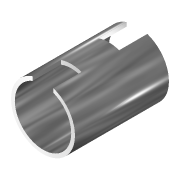
# Autodesk Inventor part: Pernament magnet
Saved by Autodesk Inventor 2020.3 (Build 243373010, 373A)
## iProperties
Created: 2021-04-26
Part Number: Pernament magnet
Material: Stainless Steel AISI 304
Document SubType Name: Modeling
Designer: marti
Density: 8 g/cm^3
Appearance: Chrome - Satin
Author: marti
Autodesk Inventor part; units mm, degrees
ref_plane "YZ Plane" through (0, 0, 0) normal (1, 0, 0) x (0, 1, 0)
ref_plane "XZ Plane" through (0, 0, 0) normal (0, 1, 0) x (-1, 0, 0)
ref_plane "XY Plane" through (0, 0, 0) normal (0, 0, 1) x (1, 0, 0)
sketch "Sketch1" plane through (0, 0, 0) normal (0, 0, 1) x (1, 0, 0)
  circle A0 centre (0, 0) radius 7.5
  circle A1 centre (0, 0) radius 8.5
  dimension "d0" = 15
  dimension "d1" = 17
  constraints: 2 centre point, 2 coincident
  measures "d0" diameter of A0
  measures "d1" diameter of A1
extrude "Extrusion1" add sketch "Sketch1" against normal mid plane 25
sketch "Sketch2" plane through (0, 0, 12.5) normal (0, 0, 1) x (1, 0, 0)
  line L0 (-2.75, 9.35) -> (-2.75, 6.9776)
  arc A0 (-2.25, 9.85) -> (-2.75, 9.35) centre (-2.25, 9.35) ccw
  line L1 (2.25, 9.85) -> (-2.25, 9.85)
  arc A1 (2.75, 9.35) -> (2.25, 9.85) centre (2.25, 9.35) ccw
  line L2 (2.75, 6.9776) -> (2.75, 9.35)
  circle A2 centre (0, 0) radius 8.5 projected
  circle A3 centre (0, 0) radius 7.5 projected
  line L3 (-2.75, 6.9776) -> (2.75, 6.9776)
  constraints: 8 end point, 6 point on circle, 2 centre point, 1 horizontal
extrude "Extrusion2" cut sketch "Sketch2" against normal blind 7.5 contours A0 L1 A1 L2 A2 L0 | A2 L2 A3 L0 | A3 L3 picked at (1.6937, 7.9533) picked at (-0.4665, 7.1078)
mirror "Mirror1" about plane through (0, 0, 0) normal (0, 0, 1) of "Extrusion2"
body "Solid1"
